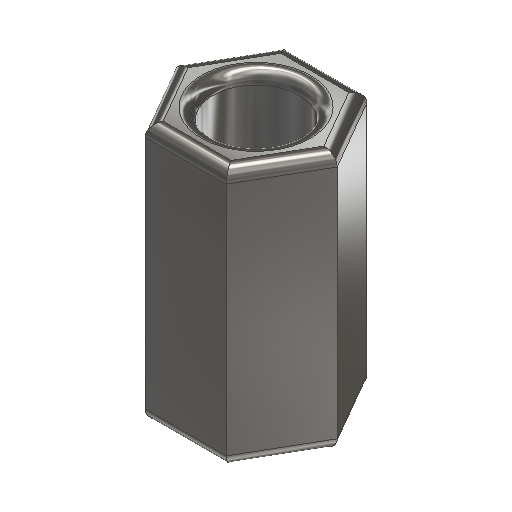
# Autodesk Inventor part: COTS_GENERIC_Z_Axis_M6_Screw_Nut
Saved by Autodesk Inventor 2026.1 (Build 301233000, 233)
## iProperties
Created: 2017-05-28
Part Number: COTS_GENERIC_Z_Axis_M6_Screw_Nut
Material: Ogólny
Document SubType Name: Modeling
Designer: Andrzej
Density: 1 g/cm^3
Appearance: Stal - polerowana
Mass: 0.973706 g
Surface Area: 10.2384 cm^2
Volume: 0.973706 cm^3
Author: Andrzej
Autodesk Inventor part; units mm, degrees
ref_plane "YZ Plane" through (0, 0, 0) normal (1, 0, 0) x (0, 1, 0)
ref_plane "XZ Plane" through (0, 0, 0) normal (0, 1, 0) x (-1, 0, 0)
ref_plane "XY Plane" through (0, 0, 0) normal (0, 0, 1) x (1, 0, 0)
sketch "Szkic1" plane through (0, 0, 0) normal (0, 0, 1) x (1, 0, 0)
  circle A0 centre (0, 0) radius 4.9
  line L0 (2.829, 4.9) -> (5.658, 0)
  line L1 (5.658, 0) -> (2.829, -4.9)
  line L2 (2.829, -4.9) -> (-2.829, -4.9)
  line L3 (-2.829, -4.9) -> (-5.658, 0)
  line L4 (-5.658, 0) -> (-2.829, 4.9)
  line L5 (-2.829, 4.9) -> (2.829, 4.9)
  circle A1 centre (0, 0) radius 3
  point P0 (0, 4.9)
  dimension "d0" = 9.8
  dimension "d1" = 6
  constraints: 12 end point, 3 coincident, 1 centre point, 1 midpoint, 1 vertical alignment, 15 other
  measures "d1" diameter of A1
extrude "Wyciągnięcie proste1" add sketch "Szkic1" along normal blind 18
fillet "Zaokrąglenie1" radius 0.8 16 edges at (1.4145, 4.9, 18) (-1.4145, 4.9, 18) (4.2435, 2.45, 18) (4.2435, -2.45, 18) (0, -4.9, 18) (-4.2435, -2.45, 18) (-4.2435, 2.45, 18) (1.4145, 4.9, 0) (-1.4145, 4.9, 0) (4.2435, 2.45, 0) (4.2435, -2.45, 0) (0, -4.9, 0) (-4.2435, -2.45, 0) (-4.2435, 2.45, 0) (-3, 0, 18) (-3, 0, 0)
